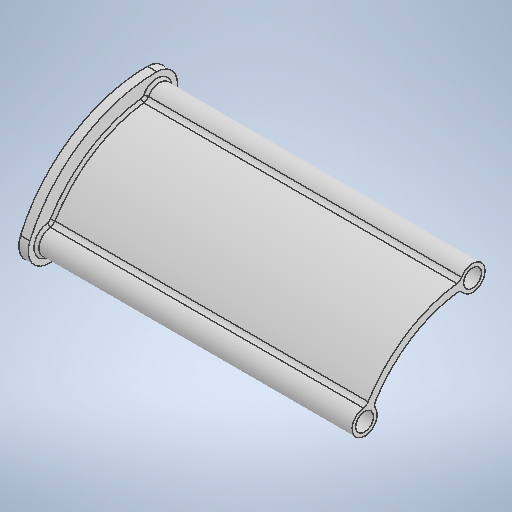
# Autodesk Inventor part: Mechanische_Anschlaege
Saved by Autodesk Inventor 2026.2 (Build 302298000, 298)
## iProperties
Created: 2026-03-24
Part Number: Mechanische_Anschlaege
Material: Generic
Document SubType Name: Modeling
Designer: Paco Ariel
Density: 1 g/cm^3
Appearance: Default
Author: Paco Ariel
Autodesk Inventor part; units mm, degrees
ref_plane "YZ Plane" through (0, 0, 0) normal (1, 0, 0) x (0, 1, 0)
ref_plane "XZ Plane" through (0, 0, 0) normal (0, 1, 0) x (-1, 0, 0)
ref_plane "XY Plane" through (0, 0, 0) normal (0, 0, 1) x (1, 0, 0)
sketch "Sketch1" plane through (0, 0, 0) normal (1, 0, 0) x (0, 1, 0)
  arc A0 (37.5, 0) -> (15.0255, 34.3582) centre (0, 0) ccw
  circle A1 centre (15.0255, 34.3582) radius 4
  circle A2 centre (37.5, 0) radius 4
  arc A3 (33.5, 0) -> (13.4227, 30.6933) centre (0, 0) ccw
  arc A4 (41.5, 0) -> (16.6282, 38.0231) centre (0, 0) ccw
  arc A5 (30.9, 0) -> (44.1, 0) centre (37.5, 0) ccw
  arc A6 (17.6699, 40.4052) -> (12.381, 28.3112) centre (15.0255, 34.3582) ccw
  arc A7 (30.9, 0) -> (12.381, 28.3112) centre (0, 0) ccw
  arc A8 (44.1, 0) -> (17.6699, 40.4052) centre (0, 0) ccw
  circle A9 centre (37.5, 0) radius 1.25
  circle A10 centre (15.051, 34.347) radius 1.25
  arc A11 (36.0575, 3.7308) -> (17.8657, 31.5417) centre (0, 0) ccw
  arc A12 (38.5575, 3.8577) -> (18.9837, 33.7814) centre (0, 0) ccw
  dimension "d2" = 8
  dimension "d3" = 8
  dimension "d4" = 83
  dimension "d7" = 13.2
  dimension "d8" = 13.2
  dimension "d9" = 88.2
  dimension "d15" = 2.5
  dimension "d16" = 2.5
  dimension "d17" = 77.5
  constraints: 27 point on circle, 13 centre point, 12 coincident, 3 tangent
  measures "d2" diameter of A1
  measures "d3" diameter of A2
  measures "d4" diameter of A4
  measures "d7" diameter of A5
  measures "d8" diameter of A6
  measures "d9" diameter of A8
  measures "d15" diameter of A9
  measures "d16" diameter of A10
  measures "d17" diameter of A12
extrude "Extrusion1" add sketch "Sketch1" along normal blind 100.5 contours A2 A11 A1 A0 | A0 A1 A12 A2 | A2 | A1 | A9 | A10
extrude "Extrusion2" add sketch "Sketch1" against normal blind 3 contours A2 A11 A1 A0 | A0 A1 A12 A2 | A2 | A1 | A12 A1 A4 A2 | A2 A3 A1 A11 | A7 A6 A8 A5 | A9 | A10
fillet "Fillet1" radius 2 4 edges at (50.25, 36.0575, 3.7308) (50.25, 17.8657, 31.5417) (50.25, 18.9837, 33.7814) (50.25, 38.5575, 3.8577)
chamfer "Chamfer2" distance 0.8 angle 45 8 edges at (0, 37.7692, -3.9909) (0, 38.7564, 4.1228) (0, 32.4284, 21.2122) (0, 19.3063, 33.8574) (0, 11.4768, 36.204) (0, 18.0284, 31.1429) (0, 30.3363, 19.8437) (0, 35.7573, 4.0397)
sketch "Sketch2" plane through (100.5, 0, 0) normal (1, 0, 0) x (0, 0, -1)
  arc A0 (-34.7347, 19.0077) -> (-30.8815, 17.0036) centre (-34.3582, 15.0255) ccw projected
  arc A1 (-3.2054, 35.1072) -> (-3.4977, 39.4406) centre (0, 37.5) ccw projected
  circle A2 centre (-34.3582, 15.0255) radius 3.75
  circle A3 centre (0, 37.5) radius 3.75
  point P0 (0, 0)
  dimension "d22" = 7.5
  dimension "d23" = 7.5
  constraints: 2 centre point, 2 coincident
  measures "d22" diameter of A2
  measures "d23" diameter of A3
extrude "Extrusion3" [suppressed]
sketch "Sketch3" plane through (102.8, 15.0255, 34.3582) normal (1, 0, 0) x (0, 0, -1)
  circle A0 centre (0, 0) radius 3.75 projected
  circle A1 centre (0, 0) radius 4
  circle A2 centre (34.3582, 22.4745) radius 3.75 projected
  circle A3 centre (34.3582, 22.4745) radius 4
  point P0 (34.3582, -15.0255)
  dimension "d26" = 8
  dimension "d27" = 8
  constraints: 2 centre point, 2 coincident
  measures "d26" diameter of A1
  measures "d27" diameter of A3
extrude "Extrusion4" [suppressed]
chamfer "Chamfer3" [suppressed]
sketch "Sketch4" plane through (104.8, 15.0255, 34.3582) normal (1, 0, 0) x (0, 0, -1)
  circle A0 centre (34.3582, 22.4745) radius 2.5 projected
  circle A1 centre (0, 0) radius 2.5 projected
  arc A2 (34.3582, 22.4745) -> (0, 0) centre (34.3582, -15.0255) ccw
  line L0 (8.4634, -2.6098) -> (-7.662, 4.4422)
  line L1 (-7.662, 4.4422) -> (-8.4634, 2.6098)
  line L2 (-8.4634, 2.6098) -> (7.662, -4.4422)
  line L3 (7.662, -4.4422) -> (8.4634, -2.6098)
  line L4 (8.4634, -2.6098) -> (-8.4634, 2.6098) construction
  line L5 (-7.662, 4.4422) -> (7.662, -4.4422) construction
  line L6 (33.3582, 13.6745) -> (33.3582, 31.2745)
  line L7 (33.3582, 31.2745) -> (35.3582, 31.2745)
  line L8 (35.3582, 31.2745) -> (35.3582, 13.6745)
  line L9 (35.3582, 13.6745) -> (33.3582, 13.6745)
  line L10 (33.3582, 13.6745) -> (35.3582, 31.2745) construction
  line L11 (33.3582, 31.2745) -> (35.3582, 13.6745) construction
  point P0 (34.3582, -15.0255)
  point P1 (0, 0)
  dimension "d33" = 37.5
  dimension "d34" = 2
  dimension "d35" = 2
  constraints: 24 end point, 4 midpoint, 4 parallel, 2 perpendicular, 2 point on circle, 1 centre point, 4 other
  measures "d33" radius of A2
  measures "d34" distance of L1.end L0.end
  measures "d35" distance of L6.end L7.end
extrude "Extrusion5" [suppressed]
sketch "Sketch5" plane through (100.5, 0, 0) normal (1, 0, 0) x (0, 0, -1)
  arc A0 (-34.7347, 19.0077) -> (-30.8815, 17.0036) centre (-34.3582, 15.0255) ccw projected
  arc A1 (-3.2054, 35.1072) -> (-3.4977, 39.4406) centre (0, 37.5) ccw projected
  circle A2 centre (-34.3582, 15.0255) radius 2.85
  circle A3 centre (0, 37.5) radius 2.85
  point P0 (0, 0)
  dimension "d38" = 5.7
  dimension "d39" = 5.7
  constraints: 2 centre point, 2 coincident
  measures "d38" diameter of A2
  measures "d39" diameter of A3
extrude "Extrusion6" cut sketch "Sketch5" against normal blind 4
sketch "Sketch6" plane through (96.5, 15.0255, 34.3582) normal (1, 0, 0) x (0, 0, -1)
  circle A0 centre (0, 0) radius 2.85 projected
  circle A1 centre (34.3582, 22.4745) radius 2.85 projected
  circle A2 centre (0, 0) radius 2.15
  circle A3 centre (34.3582, 22.4745) radius 2.15
  point P0 (34.3582, -15.0255)
  dimension "d42" = 4.3
  dimension "d43" = 4.3
  constraints: 2 centre point, 2 coincident
  measures "d42" diameter of A2
  measures "d43" diameter of A3
extrude "Extrusion7" cut sketch "Sketch6" against normal blind 2 contours A2 | A3
equation "\"d23\" = d22"
equation "\"d35\" = d34"
body "Solid1"
